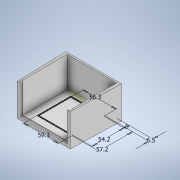
# Autodesk Inventor part: Part_C2
Saved by Autodesk Inventor 2022.6 (Build 266554010, 554A)
## iProperties
Created: 2025-05-19
Part Number: Part_C2
Material: Generic
Document SubType Name: Modeling
Designer: khinm
Density: 1 g/cm^3
Appearance: Default
Author: khinm
Autodesk Inventor part; units mm, degrees
ref_plane "YZ Plane" through (0, 0, 0) normal (1, 0, 0) x (0, 1, 0)
ref_plane "XZ Plane" through (0, 0, 0) normal (0, 1, 0) x (-1, 0, 0)
sketch "Sketch1" plane through (0, 0, 0) normal (0, 1, 0) x (-1, 0, 0)
  line L0 (47.5, -42.5) -> (-47.5, -42.5)
  line L1 (-47.5, -42.5) -> (-45, 42.5)
  line L2 (-45, 42.5) -> (45, 42.5)
  line L3 (45, 42.5) -> (47.5, -42.5)
  point P0 (0, 0)
  point P1 (0, -42.5)
  point P2 (0, 42.5)
  point P3 (46.25, 0)
  dimension "d0" = 95
  dimension "d1" = 90
  dimension "d2" = 85
  constraints: 8 end point, 3 midpoint, 2 vertical alignment, 1 horizontal, 1 horizontal alignment, 1 parallel
  measures "d0" distance of L0.start L0.end
  measures "d1" distance of L1.end L2.end
  measures "d2" distance between parallel lines of L2 L0
extrude "Extrusion1" add sketch "Sketch1" along normal mid plane 110
sketch "Sketch2" plane through (-45, 55, 42.5) normal (0, 0, 1) x (1, 0, 0)
  line L0 (3, -3) -> (87, -3)
  line L1 (87, -3) -> (87, -107)
  line L2 (87, -107) -> (3, -107)
  line L3 (3, -107) -> (3, -3)
  point P0 (45, -55)
  point P1 (3, -55)
  point P2 (45, -3)
  dimension "d5" = 84
  dimension "d6" = 104
  constraints: 8 end point, 2 midpoint, 2 parallel, 1 horizontal, 1 horizontal alignment, 1 perpendicular, 1 vertical alignment
  measures "d5" distance of L0.start L0.end
  measures "d6" distance of L0.end L1.end
extrude "Extrusion2" cut sketch "Sketch2" against normal blind 82
sketch "Sketch3" plane through (0, 55, 0) normal (0, 1, 0) x (1, 0, 0)
  line L0 (-43, -35.8) -> (43, -35.8)
  line L1 (43, -35.8) -> (43, -42.5)
  line L2 (43, -42.5) -> (-43, -42.5)
  line L3 (-43, -42.5) -> (-43, -35.8)
  line L4 (-45, -42.5) -> (45, -42.5) projected
  point P0 (0, 0)
  point P1 (0, -35.8)
  point P2 (0, -42.5)
  dimension "d10" = 86
  dimension "d12" = 6.7
  constraints: 8 end point, 2 midpoint, 2 parallel, 1 horizontal, 1 perpendicular, 1 vertical alignment
  measures "d10" distance of L0.start L0.end
  measures "d12" distance between parallel lines of L2 L0
extrude "Extrusion3" cut sketch "Sketch3" against normal blind 108.5
ref_plane "Work Plane1" through (0, 0, 42.5) normal (0, 0, 1) x (1, 0, 0)
sketch "Sketch4" plane through (0, 0, 42.5) normal (0, 0, 1) x (1, 0, 0)
  line L0 (-43, 55) -> (-43, -53.5) projected
  line L1 (43, 55) -> (43, -53.5) projected
  line L2 (-43, 55) -> (43, 55)
  line L3 (43, 55) -> (43, -53.5)
  line L4 (43, -53.5) -> (-43, -53.5)
  line L5 (-43, -53.5) -> (-43, 55)
  point P0 (0, 0)
  constraints: 8 end point, 2 parallel, 1 horizontal, 1 perpendicular
extrude "Extrusion4" add sketch "Sketch4" against normal blind 1.5
sketch "Sketch5" plane through (-45, 55, 42.5) normal (0, 0, 1) x (1, 0, 0)
  line L0 (85, -5) -> (85, -105)
  line L1 (85, -105) -> (5, -105)
  line L2 (5, -105) -> (5, -5)
  line L3 (0, 0) -> (90, 0) projected
  line L4 (0, 0) -> (0, -110) projected
  line L5 (10, -5) -> (10, 0)
  line L6 (80, -5) -> (80, 0)
  line L7 (5, -5) -> (10, -5)
  line L8 (80, -5) -> (85, -5)
  line L9 (90, -110) -> (90, 0) projected
  point P0 (45, -55)
  point P1 (45, -5)
  point P2 (5, -55)
  point P3 (80, -2.5)
  point P4 (10, -2.5)
  point P5 (7.5, -5)
  point P6 (82.5, -5)
  dimension "d20" = 5
  dimension "d21" = 5
  dimension "d22" = 10
  dimension "d23" = 10
  dimension "d24" = 5
  dimension "d25" = 5
  constraints: 14 end point, 5 midpoint, 4 parallel, 3 perpendicular, 2 horizontal, 2 point on line, 1 horizontal alignment, 1 vertical alignment
  measures "d20" distance between parallel lines of L4 L2
  measures "d21" distance between parallel lines of L0 L9
  measures "d22" distance from line of L9 point (80, -2.5)
  measures "d23" distance from line of point (10, -2.5) L4
  measures "d24" distance from line of L3 point (7.5, -5)
  measures "d25" distance from line of L3 point (82.5, -5)
extrude "Extrusion5" cut sketch "Sketch5" against normal up to surface (1.5 mm away)
sketch "Sketch6" plane through (-42, -52, -39.5) normal (0, 1, 0) x (1, 0, 0)
  line L0 (13.85, -8) -> (70.15, -8)
  line L1 (70.15, -8) -> (70.15, -62.2)
  line L2 (70.15, -62.2) -> (13.85, -62.2)
  line L3 (13.85, -62.2) -> (13.85, -8)
  line L4 (84, 0) -> (0, 0) projected
  point P0 (42, -39.5)
  point P1 (42, -8)
  dimension "d28" = 8
  dimension "d29" = 56.3
  dimension "d30" = 54.2
  constraints: 8 end point, 2 parallel, 1 horizontal, 1 midpoint, 1 perpendicular, 1 vertical alignment
  measures "d28" distance between parallel lines of L4 L0
  measures "d29" distance of L0.start L0.end
  measures "d30" distance of L0.end L1.end
sketch "Sketch7" plane through (-42, -52, -39.5) normal (0, 1, 0) x (1, 0, 0)
  line L0 (12.35, -6.5) -> (71.65, -6.5)
  line L1 (71.65, -6.5) -> (71.65, -63.7)
  line L2 (71.65, -63.7) -> (12.35, -63.7)
  line L3 (12.35, -63.7) -> (12.35, -6.5)
  line L4 (84, 0) -> (0, 0) projected
  point P0 (42, -39.5)
  point P1 (42, -6.5)
  dimension "d31" = 6.5
  dimension "d33" = 59.3
  dimension "d34" = 57.2
  constraints: 8 end point, 2 parallel, 1 horizontal, 1 midpoint, 1 perpendicular, 1 vertical alignment
  measures "d31" distance between parallel lines of L4 L0
  measures "d33" distance of L1.end L2.end
  measures "d34" distance of L0.end L1.end
body "Solid1"
